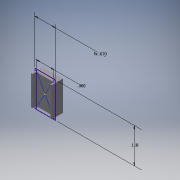
# Autodesk Inventor part: probe_carrier_nn32
Saved by Autodesk Inventor 2016 (Build 200138000, 138)
## iProperties
Created: 2016-06-26
Part Number: probe_carrier_nn32
Material: Generic
Document SubType Name: Modeling
Designer: GentnerLab
Density: 1 g/cm^3
Appearance: Default
Author: GentnerLab
Autodesk Inventor part; units mm, degrees
ref_plane "YZ Plane" through (0, 0, 0) normal (1, 0, 0) x (0, 1, 0)
ref_plane "XZ Plane" through (0, 0, 0) normal (0, 1, 0) x (-1, 0, 0)
ref_plane "XY Plane" through (0, 0, 0) normal (0, 0, 1) x (1, 0, 0)
sketch "Sketch2" plane through (0, 0, 0) normal (0, 0, 1) x (1, 0, 0)
  line L0 (-0.889, -1.5) -> (0.889, -1.5)
  line L1 (0.889, -1.5) -> (0.889, 1.5)
  line L2 (0.889, 1.5) -> (-0.889, 1.5)
  line L3 (-0.889, 1.5) -> (-0.889, -1.5)
  line L4 (-0.889, -1.5) -> (0.889, 1.5) construction
  line L5 (0.889, -1.5) -> (-0.889, 1.5) construction
  line L6 (-0.762, -1.5) -> (0.762, -1.5)
  line L7 (0.762, -1.5) -> (0.762, 1.5)
  line L8 (0.762, 1.5) -> (-0.762, 1.5)
  line L9 (-0.762, 1.5) -> (-0.762, -1.5)
  line L10 (-0.762, -1.5) -> (0.762, 1.5) construction
  line L11 (0.762, -1.5) -> (-0.762, 1.5) construction
  point P0 (0, 0)
  dimension "d0" = 3
  dimension "d1" = 1.778
  dimension "d6" = 1.524
  constraints: 24 end point, 4 midpoint, 4 parallel, 2 horizontal, 2 perpendicular, 1 point on line
  measures "d0" distance between parallel lines of L0 L2
  measures "d1" distance between parallel lines of L1 L3
  measures "d6" distance between parallel lines of L7 L9
extrude "Extrusion1" add sketch "Sketch2" against normal blind 0.635
extrude "Extrusion2" add sketch "Sketch2" along normal blind 0.3175 contours L3 L2 L9 L0 | L7 L2 L1 L0
body "Solid1"
